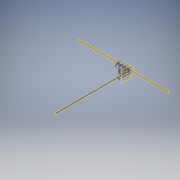
# Autodesk Inventor part: verticle connnector
Saved by Autodesk Inventor 2016 (Build 200138000, 138)
## iProperties
Created: 2016-05-26
Part Number: verticle connnector
Material: Generic
Document SubType Name: Modeling
Designer: Scott
Density: 1 g/cm^3
Appearance: Default
Author: Scott
Autodesk Inventor part; units mm, degrees
ref_plane "YZ Plane" through (0, 0, 0) normal (1, 0, 0) x (0, 1, 0)
ref_plane "XZ Plane" through (0, 0, 0) normal (0, 1, 0) x (-1, 0, 0)
ref_plane "XY Plane" through (0, 0, 0) normal (0, 0, 1) x (1, 0, 0)
ref_plane "Work Plane1" through (0, -640.4, 0) normal (0, 0, 1) x (1, 0, 0)
sketch "Sketch1" plane through (0, -640.4, 0) normal (0, 0, 1) x (1, 0, 0)
  line L0 (-438.15, 20) -> (438.15, 20) projected
  line L1 (-438.15, 0) -> (-438.15, 20) projected
  line L2 (438.15, 0) -> (-438.15, 0) projected
  line L3 (438.15, 20) -> (438.15, 0) projected
  line L4 (63.5, 20) -> (-63.5, 20)
  line L5 (-63.5, 20) -> (-63.5, 0)
  line L6 (-63.5, 0) -> (63.5, 0)
  line L7 (63.5, 0) -> (63.5, 20)
  line L8 (63.5, 20) -> (-63.5, 0) construction
  line L9 (-63.5, 20) -> (63.5, 0) construction
  point P0 (0, 640.4)
  point P1 (0, 10)
  dimension "d0" = 127
  constraints: 12 end point, 2 midpoint, 2 parallel, 1 horizontal, 1 perpendicular, 1 point on line
  measures "d0" distance of L6.end L5.end
extrude "Extrusion1" add sketch "Sketch1" along normal blind 5.08 contours L0 L7 L2 L5
sketch "Sketch2" plane through (-63.5, -640.4, 0) normal (0, -1, 0) x (1, 0, 0)
  line L0 (501.65, 0) -> (-374.65, 0) projected
  line L1 (-374.65, -20) -> (-374.65, 0) projected
  line L2 (501.65, -20) -> (-374.65, -20) projected
  line L3 (501.65, 0) -> (501.65, -20) projected
  line L4 (0, 5.08) -> (127, 5.08) projected
  line L5 (0, 5.08) -> (127, 5.08)
  line L6 (127, 5.08) -> (127, -20)
  line L7 (127, -20) -> (0, -20)
  line L8 (0, -20) -> (0, 5.08)
  point P0 (63.5, 0)
  constraints: 8 end point, 2 parallel, 1 horizontal, 1 perpendicular, 1 point on line
extrude "Extrusion2" add sketch "Sketch2" along normal blind 5.08 contours L6 L2 L8 L0 | L0 L8 L4 L6
ref_plane "Work Plane2" through (1.9201, -666.48, -20) normal (0, 0, -1) x (-1, 0, 0)
sketch "Sketch3" plane through (1.9201, -666.48, -20) normal (0, 0, -1) x (-1, 0, 0)
  line L0 (21, -21) -> (-21, -21)
  line L1 (-21, -21) -> (-21, 21)
  line L2 (-21, 21) -> (21, 21)
  line L3 (21, 21) -> (21, -21)
  line L4 (21, -21) -> (-21, 21) construction
  line L5 (-21, -21) -> (21, 21) construction
  line L6 (65.4201, 26.08) -> (-61.5799, 26.08) projected
  line L7 (26.08, -26.08) -> (-26.08, -26.08)
  line L8 (-26.08, -26.08) -> (-26.08, 26.08)
  line L9 (-26.08, 26.08) -> (26.08, 26.08)
  line L10 (26.08, 26.08) -> (26.08, -26.08)
  line L11 (26.08, -26.08) -> (-26.08, 26.08) construction
  line L12 (-26.08, -26.08) -> (26.08, 26.08) construction
  line L13 (21, -21) -> (26.08, -21)
  line L14 (21, 21) -> (26.08, 21)
  line L15 (-61.5799, 21) -> (65.4201, 21) projected
  point P0 (1.9201, 666.48)
  point P1 (0, 0)
  point P2 (0, 0)
  dimension "d5" = 42
  dimension "d6" = 42
  constraints: 28 end point, 5 midpoint, 5 point on line, 4 parallel, 3 perpendicular, 2 horizontal
  measures "d5" distance of L1.end L2.end
  measures "d6" distance of L0.end L1.end
extrude "Extrusion3" add sketch "Sketch3" against normal blind 47 contours L13 L10 L7 L8 L15 L1 L0 | L2 L15 L8 L6 L10 L14
sketch "Sketch4" plane through (1.9201, -666.48, 27) normal (0, 0, 1) x (1, 0, 0)
  line L0 (26.08, 21) -> (26.08, -26.08) projected
  line L1 (-26.08, 26.08) -> (26.08, 26.08)
  line L2 (26.08, 26.08) -> (26.08, -26.08)
  line L3 (26.08, -26.08) -> (-26.08, -26.08)
  line L4 (-26.08, -26.08) -> (-26.08, 26.08)
  line L5 (-26.08, 26.08) -> (26.08, -26.08) construction
  line L6 (26.08, 26.08) -> (-26.08, -26.08) construction
  circle A0 centre (0, 0) radius 12.5
  line L7 (0, 0) -> (0, 15.5)
  line L8 (0, 0) -> (15.5, 0) construction
  line L9 (0, 15.5) -> (15.5, 15.5)
  circle A1 centre (15.5, 15.5) radius 2
  circle A2 centre (15.5, -15.5) radius 2
  circle A3 centre (-15.5, -15.5) radius 2
  circle A4 centre (-15.5, 15.5) radius 2
  point P0 (-1.9201, 666.48)
  dimension "d9" = 25
  dimension "d10" = 15.5
  dimension "d11" = 90
  dimension "d12" = 15.5
  dimension "d13" = 4
  dimension "d14" = 4
  dimension "d15" = 4
  dimension "d16" = 4
  constraints: 18 end point, 5 centre point, 4 point on line, 2 coincident, 2 horizontal, 2 midpoint, 2 parallel, 2 perpendicular, 1 vertical
  measures "d9" diameter of A0
  measures "d10" distance of L7.start L7.end
  measures "d11" angle of L8 L7
  measures "d12" distance of L7.end L9.end
  measures "d13" diameter of A1
  measures "d14" diameter of A2
  measures "d15" diameter of A3
  measures "d16" diameter of A4
extrude "Extrusion4" add sketch "Sketch4" along normal blind 5.08
sketch "Sketch5" plane through (-63.5, -645.48, 0) normal (0, -1, 0) x (1, 0, 0)
  line L0 (91.5001, 742) -> (91.5001, -20) projected
  line L1 (111.5001, 742) -> (91.5001, 742) projected
  line L2 (111.5001, -20) -> (111.5001, 742) projected
  line L3 (91.5001, -20) -> (111.5001, -20) projected
  line L4 (91.5001, 67.9979) -> (111.5001, 67.9979)
  line L5 (127, 5.08) -> (0, 5.08) projected
  line L6 (111.5001, 67.9979) -> (127, 5.08)
  line L7 (127, -20) -> (127, 5.08) projected
  line L8 (127, 5.08) -> (127, -20)
  line L9 (91.5001, 5.08) -> (91.5001, -20) projected
  line L10 (127, -20) -> (91.5001, -20)
  line L11 (91.5001, -20) -> (91.5001, 67.9979)
  point P0 (63.5, 0)
  constraints: 10 end point, 2 collinear, 2 perpendicular, 2 point on line
extrude "Extrusion5" add sketch "Sketch5" against normal blind 5.08 contours L4 L2 L5 L0 | L5 L2 L3 L0 | L6 L5 L2 | L5 L7 L10 L2
sketch "Sketch6" plane through (0, -640.4, 5.08) normal (0, 0, 1) x (1, 0, 0)
  line L0 (-24.1599, 0) -> (63.5, 0) projected
  line L1 (63.5, 20) -> (63.5, 0) projected
  line L2 (63.5, 20) -> (-63.5, 20) projected
  line L3 (-63.5, 20) -> (-63.5, -5.08) projected
  line L4 (-24.1599, -5.08) -> (-63.5, -5.08) projected
  line L5 (-24.1599, -5.08) -> (-24.1599, 0) projected
  circle A0 centre (53.34, 10) radius 2.5
  circle A1 centre (21.59, 10) radius 2.5
  circle A2 centre (-10.16, 10) radius 2.5
  circle A3 centre (-41.91, 10) radius 2.5
  point P0 (0, 640.4)
  dimension "d21" = 5
  dimension "d22" = 5
  dimension "d23" = 5
  dimension "d24" = 5
  dimension "d25" = 10.16
  dimension "d26" = 31.75
  dimension "d27" = 31.75
  dimension "d28" = 31.75
  constraints: 4 centre point
  measures "d21" diameter of A0
  measures "d22" diameter of A1
  measures "d23" diameter of A2
  measures "d24" diameter of A3
  measures "d25" distance from line of L1 A0.centre
  measures "d26" distance of A1.centre A0.centre
  measures "d27" distance of A1.centre A2.centre
  measures "d28" distance of A2.centre A3.centre
extrude "Extrusion6" cut sketch "Sketch6" against normal blind 50.8 contours A0 | A1 | A2 | A3
sketch "Sketch7" plane through (-24.1599, -640.4, 32.08) normal (0, 1, 0) x (1, 0, 0)
  line L0 (0, 27) -> (87.6599, 27) projected
  line L1 (0, 27) -> (0, 0) projected
  line L2 (52.16, 0) -> (0, 0) projected
  line L3 (52.16, 0) -> (52.16, -35.9179) projected
  line L4 (52.16, -35.9179) -> (72.16, -35.9179) projected
  line L5 (72.16, -35.9179) -> (87.6599, 27) projected
  circle A0 centre (62.16, -25.7579) radius 2.5
  circle A1 centre (62.16, -6.7079) radius 2.5
  circle A2 centre (62.16, 18.6921) radius 2.5
  point P0 (24.1599, 32.08)
  dimension "d31" = 5
  dimension "d32" = 5
  dimension "d33" = 5
  dimension "d34" = 10.16
  dimension "d35" = 19.05
  dimension "d36" = 25.4
  constraints: 3 centre point
  measures "d31" diameter of A0
  measures "d32" diameter of A1
  measures "d33" diameter of A2
  measures "d34" distance from line of L4 A0.centre
  measures "d35" distance of A0.centre A1.centre
  measures "d36" distance of A2.centre A1.centre
extrude "Extrusion7" cut sketch "Sketch7" against normal blind 50.8 contours A0 | A1 | A2
sketch "Sketch8" plane through (-63.5, -620.4, 0) normal (0, 1, 0) x (1, 0, 0)
  line L0 (127, 0) -> (0, 0) projected
  line L1 (0, 0) -> (0, -5.08) projected
  line L2 (127, -5.08) -> (0, -5.08) projected
  line L3 (127, 0) -> (127, -5.08) projected
  line L4 (127, 0) -> (127, -5.08) projected
  line L5 (0, 20) -> (127, 20) projected
  line L6 (127, -5.08) -> (0, -5.08)
  line L7 (0, -5.08) -> (0, 20)
  line L8 (0, 20) -> (127, 20)
  line L9 (127, 20) -> (127, -5.08)
  point P0 (63.5, 0)
  constraints: 8 end point, 2 parallel, 1 horizontal, 1 perpendicular
extrude "Extrusion8" add sketch "Sketch8" along normal blind 5.08
sketch "Sketch9" plane through (-63.5, -615.32, 0) normal (0, 1, 0) x (1, 0, 0)
  line L0 (24.09, -5.08) -> (19.09, -5.08) projected
  line L1 (55.84, -5.08) -> (50.84, -5.08) projected
  line L2 (87.59, -5.08) -> (82.59, -5.08) projected
  line L3 (119.34, -5.08) -> (114.34, -5.08) projected
  line L4 (127, -5.08) -> (127, 20) projected
  line L5 (127, 20) -> (0, 20) projected
  line L6 (0, 20) -> (0, -5.08) projected
  line L7 (0, -5.08) -> (127, -5.08) projected
  circle A0 centre (21.59, 7.46) radius 2.5
  circle A1 centre (53.34, 7.46) radius 2.5
  circle A2 centre (86.4201, 7.46) radius 2.5
  circle A3 centre (116.84, 7.46) radius 2.5
  point P0 (63.5, 0)
  dimension "d41" = 5
  dimension "d42" = 5
  constraints: 4 centre point
  measures "d41" diameter of A2
  measures "d42" diameter of A3
extrude "Extrusion9" cut sketch "Sketch9" against normal blind 5.08 contours A0 | A1 | A2 | A3
ref_plane "Work Plane3" through (1.3449, -715.5816, 32.08) normal (0, 0, -1) x (-1, 0, 0)
sketch "Sketch10" plane through (63.5, -640.4, -20) normal (0, 0, -1) x (-1, 0, 0)
  line L0 (35.4999, -5.08) -> (35.4999, -52.16) projected
  line L1 (35.4999, -52.16) -> (87.6599, -52.16) projected
  line L2 (87.6599, -52.16) -> (87.6599, -47.08) projected
  line L3 (87.6599, -47.08) -> (40.5799, -47.08) projected
  line L4 (40.5799, -47.08) -> (40.5799, -5.08) projected
  line L5 (127, -5.08) -> (40.5799, -5.08) projected
  line L6 (127, 0) -> (127, -5.08) projected
  line L7 (127, 0) -> (0, 0) projected
  line L8 (0, 0) -> (0, -5.08) projected
  line L9 (35.4999, -5.08) -> (0, -5.08) projected
  circle A0 centre (62.1551, -75.1816) radius 4 projected
  circle A1 centre (61.5799, -26.08) radius 12.5 projected
  arc A2 (54.2117, -80.4378) -> (70.2939, -80.1299) centre (62.1551, -75.1816) ccw
  line L10 (87.6599, -52.16) -> (87.6599, -47.08) projected
  line L11 (70.1999, -80.2813) -> (87.6599, -52.16)
  line L12 (35.4999, -52.16) -> (54.2117, -80.4378)
  line L13 (35.4999, -5.08) -> (35.4999, -52.16) projected
  line L14 (87.6599, -52.16) -> (35.4999, -52.16)
  point P0 (63.5, 640.4)
  dimension "d45" = 19.05
  constraints: 6 end point, 3 point on circle, 1 centre point, 1 coincident, 1 perpendicular, 1 point on line, 1 tangent
  measures "d45" diameter of A2
extrude "Extrusion10" add sketch "Sketch10" against normal blind 76.2 contours L1 L11 A2 L12
sketch "Sketch11" plane through (-24.1599, -645.48, 5.08) normal (-1, 0, 0) x (0, 0, 1)
  line L0 (27, -47.08) -> (51.12, -47.08) projected
  line L1 (51.12, -75.3578) -> (51.12, -47.08) projected
  line L2 (51.12, -61.2189) -> (27, -47.08)
  line L3 (51.12, -61.2189) -> (51.12, -47.08)
  point P0 (-5.08, 645.48)
  constraints: 4 end point, 1 collinear, 1 midpoint
extrude "Extrusion11" cut sketch "Sketch11" against normal blind 76.2
ref_plane "Work Plane4" through (1.3449, -715.5816, 32.08) normal (0, 0, -1) x (-1, 0, 0)
sketch "Sketch12" plane through (1.3449, -715.5816, 32.08) normal (0, 0, -1) x (-1, 0, 0)
  circle A0 centre (0, 0) radius 4 projected
  circle A1 centre (0, 0) radius 4
  point P0 (1.3449, 715.5816)
  constraints: 1 centre point, 1 coincident
extrude "Extrusion12" add sketch "Sketch12" along normal up to surface (52.08 mm away)
sketch "Sketch13" plane through (-63.5, -645.48, 0) normal (0, -1, 0) x (1, 0, 0)
  line L0 (39.3401, 5.08) -> (0, 5.08) projected
  line L1 (39.3401, -20) -> (39.3401, 32.08) projected
  line L2 (39.3401, 5.08) -> (0, 5.08)
  line L3 (0, 5.08) -> (0, 32.08)
  line L4 (0, 32.08) -> (39.3401, 32.08)
  line L5 (39.3401, 32.08) -> (39.3401, 5.08)
  point P0 (63.5, 0)
  constraints: 8 end point, 2 parallel, 1 horizontal, 1 perpendicular
extrude "Extrusion13" add sketch "Sketch13" against normal blind 5.08
sketch "Sketch14" plane through (-63.5, -640.4, -20) normal (-1, 0, 0) x (0, 0, 1)
  line L0 (20, 20) -> (20, 0) projected
  line L1 (20, 0) -> (0, 0) projected
  line L2 (0, 0) -> (0, -5.08) projected
  line L3 (0, -5.08) -> (52.08, -5.08) projected
  line L4 (52.08, -5.08) -> (52.08, 0) projected
  line L5 (25.08, 0) -> (52.08, 0) projected
  line L6 (25.08, 0) -> (25.08, 25.08) projected
  line L7 (0, 25.08) -> (25.08, 25.08) projected
  line L8 (0, 20) -> (0, 25.08) projected
  line L9 (0, 20) -> (20, 20) projected
  line L10 (25.08, 0) -> (25.08, 25.08) projected
  line L11 (52.08, 0) -> (25.08, 25.08)
  line L12 (25.08, 25.08) -> (25.08, 0)
  line L13 (25.08, 0) -> (52.08, 0) projected
  line L14 (25.08, 0) -> (52.08, 0)
  point P0 (20, 640.4)
  constraints: 6 end point, 2 collinear
extrude "Extrusion14" add sketch "Sketch14" against normal blind 5.08 contours L11 L5 L6
ref_plane "Work Plane5" through (-26.9875, -640.4, -20) normal (-1, 0, 0) x (0, 0, 1)
ref_plane "Work Plane6" through (6.35, -640.4, -20) normal (-1, 0, 0) x (0, 0, 1)
sketch "Sketch15" plane through (-26.9875, -640.4, -20) normal (-1, 0, 0) x (0, 0, 1)
  line L0 (25.08, 0) -> (52.08, 0) projected
  line L1 (25.0542, -0.4281) -> (25.0599, 5.7289) projected
  line L2 (25.0599, 5.7289) -> (25.1096, 59.7039) projected
  line L3 (25.08, 25.08) -> (52.08, 0)
  line L4 (25.08, 0) -> (25.08, 25.08)
  line L5 (25.08, 0) -> (52.08, 0)
  point P0 (20, 640.4)
  constraints: 6 end point, 1 horizontal
extrude "Extrusion15" add sketch "Sketch15" along normal mid plane 5.08
sketch "Sketch16" plane through (6.35, -640.4, -20) normal (-1, 0, 0) x (0, 0, 1)
  line L0 (52.08, 0) -> (25.08, 0) projected
  line L1 (52.08, 0) -> (25.08, 25.08) projected
  line L2 (25.08, 0) -> (25.08, 25.08) projected
  point P0 (20, 640.4)
extrude "Extrusion16" add sketch "Sketch16" along normal mid plane 5.08
sketch "Sketch17" plane through (28.0001, -645.48, 32.08) normal (-1, 0, 0) x (0, 0, 1)
  line L0 (0, 0) -> (0, 5.08) projected
  line L1 (35.9179, 0) -> (0, 0) projected
  line L2 (35.9179, 0) -> (35.9179, 5.08) projected
  line L3 (0, 5.08) -> (35.9179, 5.08) projected
  line L4 (-32.08, 25.08) -> (-32.08, 5.08) projected
  line L5 (-32.08, 5.08) -> (-52.08, 5.08) projected
  line L6 (-52.08, 5.08) -> (-52.08, 0) projected
  line L7 (-52.08, 0) -> (0, 0) projected
  line L8 (0, 0) -> (0, 5.08) projected
  line L9 (0, 5.08) -> (-27, 30.16) projected
  line L10 (-52.08, 30.16) -> (-27, 30.16) projected
  line L11 (-52.08, 25.08) -> (-52.08, 30.16) projected
  line L12 (-52.08, 25.08) -> (-32.08, 25.08) projected
  line L13 (0, 5.08) -> (-27, 30.16) projected
  line L14 (-27, 30.16) -> (35.9179, 5.08)
  line L15 (35.9179, 0) -> (0, 0) projected
  line L16 (0, 0) -> (-27, 0)
  line L17 (-52.08, 0) -> (0, 0) projected
  line L18 (-27, 0) -> (-27, 30.16)
  point P0 (-32.08, 645.48)
  constraints: 6 end point, 1 perpendicular, 1 point on line
extrude "Extrusion17" add sketch "Sketch17" against normal blind 2.54 contours L7 L18 L9 L0 | L0 L3 L2 L1 | L9 L14 L3
ref_plane "Work Plane7" through (48.0001, -645.48, 67.9979) normal (1, 0, 0) x (0, 1, 0)
sketch "Sketch18" plane through (48.0001, -645.48, 67.9979) normal (1, 0, 0) x (0, 1, 0)
  line L0 (5.08, -62.9179) -> (5.08, 0) projected
  line L1 (30.16, -62.9179) -> (5.08, -62.9179) projected
  line L2 (30.16, -62.9179) -> (5.08, 0) projected
  point P0 (645.48, -67.9979)
extrude "Extrusion18" add sketch "Sketch18" against normal blind 2.54
sketch "Sketch19" plane through (63.5, -640.4, -20) normal (0, 0, -1) x (-1, 0, 0)
  line L0 (35.4999, -5.08) -> (35.4999, -52.16) projected
  line L1 (35.4999, -52.16) -> (54.2117, -80.4378) projected
  arc A0 (54.2117, -80.4378) -> (70.1999, -80.2813) centre (62.1551, -75.1816) ccw projected
  line L2 (70.1999, -80.2813) -> (87.6599, -52.16) projected
  line L3 (87.6599, -52.16) -> (87.6599, -47.08) projected
  line L4 (87.6599, -47.08) -> (40.5799, -47.08) projected
  line L5 (40.5799, -47.08) -> (40.5799, -5.08) projected
  line L6 (127, -5.08) -> (40.5799, -5.08) projected
  line L7 (127, 0) -> (127, -5.08) projected
  line L8 (127, 0) -> (0, 0) projected
  line L9 (0, 0) -> (0, -5.08) projected
  line L10 (35.4999, -5.08) -> (0, -5.08) projected
  line L11 (40.5799, -47.08) -> (35.4999, -47.08)
  line L12 (41.5914, -52.16) -> (81.6804, -52.16)
  line L13 (81.6804, -52.16) -> (65.899, -77.5777)
  arc A1 (58.4482, -77.6345) -> (65.899, -77.5777) centre (62.1551, -75.1816) ccw
  line L14 (58.4482, -77.6345) -> (41.5914, -52.16)
  point P0 (63.5, 640.4)
  dimension "d67" = 5.08
  constraints: 8 end point, 2 point on circle, 1 centre point, 1 horizontal, 1 point on line, 3 other
  measures "d67" distance between parallel lines of L4 L12
extrude "Extrusion19" cut sketch "Sketch19" against normal blind 45.085 contours L12 L13 A1 L14
chamfer "Chamfer1" distance 26.9875 angle 45 1 edges at (1.8641, -692.56, 25.085)
ref_plane "Work Plane8" through (28.0001, -665.48, 361) normal (0, -1, 0) x (0, 0, 1)
sketch "Sketch20" plane through (28.0001, -665.48, 361) normal (0, -1, 0) x (0, 0, 1)
  line L0 (-381, -20) -> (381, -20) projected
  line L1 (381, 0) -> (381, -20) projected
  line L2 (-381, 0) -> (381, 0) projected
  line L3 (-381, -20) -> (-381, 0) projected
  line L4 (-293.0021, 0) -> (-328.92, 0) projected
  line L5 (-381, -20) -> (-293.0021, -20)
  line L6 (-293.0021, -20) -> (-293.0021, 0)
  line L7 (-293.0021, 0) -> (-381, 0)
  line L8 (-381, 0) -> (-381, -20)
  line L9 (-328.92, 0) -> (-381, 0) projected
  line L10 (-381, 0) -> (-381, -35.4999) projected
  line L11 (-381, -35.4999) -> (-355.92, -35.4999) projected
  line L12 (-355.92, -35.4999) -> (-293.0021, -20) projected
  line L13 (-293.0021, -20) -> (-293.0021, 0) projected
  line L14 (-293.0021, 0) -> (-328.92, 0) projected
  circle A0 centre (-322.2121, -10) radius 2.5 projected
  circle A1 centre (-303.1621, -10) radius 2.5 projected
  circle A2 centre (-347.6121, -10) radius 2.5 projected
  point P0 (-361, 28.0001)
  constraints: 8 end point, 2 parallel, 1 horizontal, 1 perpendicular
extrude "Extrusion20" add sketch "Sketch20" along normal blind 5.08 contours L3 L2 L6 L0 | L0 L12 L11 L10
ref_plane "Work Plane9" through (48.0001, -665.48, 361) normal (1, 0, 0) x (0, 0, -1)
sketch "Sketch21" plane through (48.0001, -665.48, 361) normal (1, 0, 0) x (0, 0, -1)
  line L0 (381, 0) -> (355.92, 0) projected
  line L1 (355.92, 0) -> (355.92, -5.08) projected
  line L2 (381, -5.08) -> (355.92, -5.08) projected
  line L3 (381, 0) -> (381, -5.08) projected
  line L4 (361, 25.08) -> (361, 45.08) projected
  line L5 (361, 45.08) -> (381, 45.08) projected
  line L6 (381, 45.08) -> (381, 50.16) projected
  line L7 (355.92, 50.16) -> (381, 50.16) projected
  line L8 (355.92, 50.16) -> (355.92, 25.08) projected
  line L9 (355.92, 25.08) -> (355.92, 20) projected
  line L10 (381, 20) -> (355.92, 20) projected
  line L11 (381, 25.08) -> (381, 20) projected
  line L12 (381, 25.08) -> (361, 25.08) projected
  line L13 (381, -5.08) -> (355.92, -5.08) projected
  line L14 (381, 25.08) -> (381, 20) projected
  line L15 (355.92, -5.08) -> (381, -5.08)
  line L16 (381, -5.08) -> (381, 25.08)
  line L17 (381, 25.08) -> (355.92, 25.08)
  line L18 (355.92, 25.08) -> (355.92, -5.08)
  point P0 (361, 665.48)
  constraints: 8 end point, 2 parallel, 1 horizontal, 1 perpendicular
extrude "Extrusion21" add sketch "Sketch21" along normal blind 5.08 contours L0 L18 L10 L16 | L10 L9 L17 L12 L11
chamfer "Chamfer2" distance 6.35 angle 45 2 edges at (53.0801, -645.48, -7.46) (53.0801, -665.48, -7.46)
sketch "Sketch22" plane through (63.5, -640.4, -20) normal (0, 0, -1) x (-1, 0, 0)
  line L0 (35.4999, -30.16) -> (35.4999, -52.16) projected
  line L1 (0, -25.08) -> (0, -30.16) projected
  line L2 (35.4999, -52.16) -> (0, -30.16)
  line L3 (35.4999, -30.16) -> (0, -30.16) projected
  line L4 (35.4999, -52.16) -> (35.4999, -30.16)
  line L5 (35.4999, -30.16) -> (0, -30.16)
  point P0 (63.5, 640.4)
  constraints: 6 end point, 1 perpendicular, 1 vertical
extrude "Extrusion22" add sketch "Sketch22" against normal blind 5.08
sketch "Sketch23" plane through (1.9201, -666.48, 32.08) normal (0, 0, 1) x (1, 0, 0)
  line L0 (26.08, -26.08) -> (26.08, -4.08) projected
  line L1 (26.08, -4.08) -> (61.5799, -4.08) projected
  line L2 (61.5799, -4.08) -> (46.08, -4.08) projected
  line L3 (46.08, -4.08) -> (26.08, -4.08) projected
  line L4 (38.58, -4.08) -> (33.58, -4.08) projected
  line L5 (38.58, -4.08) -> (33.58, -4.08) projected
  line L6 (38.58, -4.08) -> (33.58, -4.08) projected
  line L7 (26.08, -4.08) -> (54.8744, -4.08)
  line L8 (61.5799, -4.08) -> (46.08, -4.08) projected
  line L9 (26.08, -26.08) -> (16.7241, -40.2189) projected
  line L10 (26.08, -26.08) -> (54.8744, -4.08)
  point P0 (-1.9201, 666.48)
  constraints: 4 end point, 1 point on line
extrude "Extrusion23" add sketch "Sketch23" against normal blind 5.08
chamfer "Chamfer3" distance 7.9375 angle 45 1 edges at (28.0001, -681.56, 27)
chamfer "Chamfer4" distance 7.9375 angle 45 1 edges at (28.0001, -681.56, -14.92)
sketch "Sketch24" plane through (28.0001, -665.48, 32.08) normal (-1, 0, 0) x (0, 0, 1)
  line L0 (0, 20) -> (0, 25.08) projected
  line L1 (35.9179, 20) -> (0, 20) projected
  line L2 (35.9179, 20) -> (35.9179, 25.08) projected
  line L3 (35.9179, 25.08) -> (-27, 50.16) projected
  line L4 (-27, 25.08) -> (-27, 50.16) projected
  line L5 (0, 25.08) -> (-27, 25.08) projected
  line L6 (0, -5.08) -> (0, 0) projected
  line L7 (35.9179, -5.08) -> (0, -5.08) projected
  line L8 (35.9179, 0) -> (35.9179, -5.08) projected
  line L9 (35.9179, 0) -> (0, 0) projected
  line L10 (35.9179, 25.08) -> (0, 25.08)
  line L11 (35.9179, 25.08) -> (-27, 25.08) projected
  line L12 (35.9179, 25.08) -> (0, 25.08)
  line L13 (0, 25.08) -> (0, -5.08)
  line L14 (0, -5.08) -> (35.9179, -5.08)
  line L15 (35.9179, -5.08) -> (35.9179, 25.08)
  point P0 (-32.08, 665.48)
  constraints: 10 end point, 2 parallel, 1 collinear, 1 horizontal, 1 perpendicular
extrude "Extrusion24" add sketch "Sketch24" along normal blind 2.54 contours L0 L10 L2 L1 | L1 L15 L9 L13 | L9 L8 L7 L6
sketch "Sketch25" plane through (1.9201, -666.48, 27) normal (0, 0, -1) x (-1, 0, 0)
  line L0 (-21.5, -21.5) -> (21.5, -21.5)
  line L1 (21.5, -21.5) -> (21.5, 21.5)
  line L2 (21.5, 21.5) -> (-21.5, 21.5)
  line L3 (-21.5, 21.5) -> (-21.5, -21.5)
  line L4 (-21.5, -21.5) -> (21.5, 21.5) construction
  line L5 (21.5, -21.5) -> (-21.5, 21.5) construction
  point P0 (1.9201, 666.48)
  point P1 (0, 0)
  dimension "d92" = 43
  dimension "d93" = 43
  constraints: 12 end point, 2 midpoint, 2 parallel, 1 horizontal, 1 perpendicular
  measures "d92" distance of L2.end L1.end
  measures "d93" distance of L1.end L0.end
extrude "Extrusion25" cut sketch "Sketch25" along normal blind 59.69
sketch "Sketch26" plane through (-63.5, -645.48, 0) normal (0, -1, 0) x (1, 0, 0)
  circle A0 centre (21.59, -7.46) radius 2.5 projected
  circle A1 centre (116.84, -7.46) radius 2.5 projected
  point P0 (63.5, 0)
extrude "Extrusion26" cut sketch "Sketch26" against normal blind 59.69 contours A0
body "Solid1"
